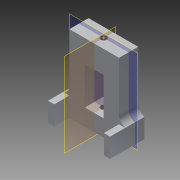
# Autodesk Inventor part: servo_attachement
Saved by Autodesk Inventor 2015 SP1 (Build 190203100, 203)
## iProperties
Created: 2015-07-14
Part Number: servo_attachement
Material: ABS Plastic
Document SubType Name: Modeling
Designer: Alexandre Cherpillod
Density: 1.06 g/cm^3
Appearance: Smooth - White
Mass: 0.981456 g
Surface Area: 9.36047 cm^2
Volume: 0.925902 cm^3
Author: Alexandre Cherpillod
Autodesk Inventor part; units mm, degrees
ref_plane "YZ Plane" through (0, 0, 0) normal (1, 0, 0) x (0, 1, 0)
ref_plane "XZ Plane" through (0, 0, 0) normal (0, 1, 0) x (-1, 0, 0)
ref_plane "XY Plane" through (0, 0, 0) normal (0, 0, 1) x (1, 0, 0)
sketch "Sketch6" plane through (0, 0, 0) normal (0, 0, 1) x (1, 0, 0)
  line L0 (-5.95, 2.3) -> (5.95, 2.3)
  line L1 (5.95, 2.3) -> (5.95, -2.3)
  line L2 (5.95, -2.3) -> (-5.95, -2.3)
  line L3 (-5.95, -2.3) -> (-5.95, 2.3)
  line L4 (-5.95, 2.3) -> (5.95, -2.3) construction
  line L5 (5.95, 2.3) -> (-5.95, -2.3) construction
  point P0 (0, 0)
  point P1 (0, 0)
  dimension "d66" = 11.9
  dimension "d67" = 4.6
  constraints: 12 end point, 2 midpoint, 2 parallel, 1 coincident, 1 horizontal, 1 perpendicular
  measures "d66" distance of L1.end L2.end
  measures "d67" distance of L0.end L1.end
extrude "Extrusion6" add sketch "Sketch6" against normal blind 18.4
hole "Hole6" at (0, 0, 0) direction (0, 0, -1) diameter 1.45 depth 7 tip angle 118
sketch "Sketch7" plane through (5.95, -2.3, 0) normal (1, 0, 0) x (0, 0, -1)
  line L0 (18.4, 4.6) -> (13.7908, 4.6)
  line L1 (13.7908, 4.6) -> (13.7908, -3.6343)
  line L2 (13.7908, -3.6343) -> (18.4, -3.6343)
  line L3 (18.4, -3.6343) -> (18.4, 4.6)
  point P0 (0, 2.3)
  constraints: 8 end point, 2 parallel, 1 horizontal, 1 perpendicular
extrude "Extrusion7" add sketch "Sketch7" along normal blind 1.5
ref_plane "Work Plane13" through (0, -2.3, 0) normal (1, 0, 0) x (0, 0, -1)
mirror "Mirror1" about plane through (0, -2.3, 0) normal (1, 0, 0) of "Extrusion7"
fillet "Fillet3" radius 2 2 edges at (5.95, 0, -13.7908) (-5.95, 0, -13.7908)
sketch "Sketch8" plane through (-5.95, 2.3, 0) normal (0, 1, 0) x (1, 0, 0)
  line L0 (3.7, 5.4) -> (8.2, 5.4)
  line L1 (8.2, 5.4) -> (8.2, 14.4)
  line L2 (8.2, 14.4) -> (3.7, 14.4)
  line L3 (3.7, 14.4) -> (3.7, 5.4)
  line L4 (3.7, 5.4) -> (8.2, 14.4) construction
  line L5 (8.2, 5.4) -> (3.7, 14.4) construction
  line L6 (5.95, 22.08) -> (5.95, -3.68) construction
  line L7 (13.4, 18.4) -> (-1.5, 18.4) projected
  point P0 (5.95, 0)
  point P1 (5.95, 9.9)
  point P2 (5.95, 9.9)
  dimension "d87" = 4
  dimension "d88" = 4.5
  dimension "d101" = 9
  constraints: 12 end point, 3 midpoint, 2 parallel, 1 horizontal, 1 perpendicular, 1 point on line
  measures "d87" distance between parallel lines of L2 L7
  measures "d88" distance between parallel lines of L1 L3
  measures "d101" distance between parallel lines of L2 L0
extrude "Extrusion8" cut sketch "Sketch8" against normal through all
ref_plane "Work Plane14" through (-5.95, 0, 0) normal (0, 1, 0) x (1, 0, 0)
hole "Hole7" at (0, 0, -18.4) direction (0, 0, 1) diameter 1.48 depth 7 tip angle 118
body "Solid4"
